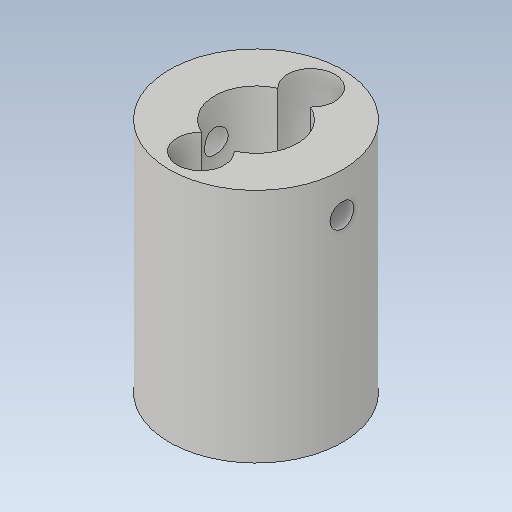
# Autodesk Inventor part: end_effector_connector_arm2_grande
Saved by Autodesk Inventor 2020.1 (Build 241239000, 239)
## iProperties
Created: 2018-02-20
Part Number: end_effector_connector_arm2_grande
Material: Generic
Document SubType Name: Modeling
Designer: Bardo91
Density: 1 g/cm^3
Appearance: Default
Author: Bardo91
Autodesk Inventor part; units mm, degrees
ref_plane "YZ Plane" through (0, 0, 0) normal (1, 0, 0) x (0, 1, 0)
ref_plane "XZ Plane" through (0, 0, 0) normal (0, 1, 0) x (-1, 0, 0)
ref_plane "XY Plane" through (0, 0, 0) normal (0, 0, 1) x (1, 0, 0)
sketch "Boceto5" plane through (0, 0, 0) normal (0, 1, 0) x (-1, 0, 0)
  circle A0 centre (0, 0) radius 11
  line L0 (0, 0) -> (0, -7)
  line L1 (0, 0) -> (0, 7)
  circle A1 centre (0, 7) radius 1.5
  circle A2 centre (0, -7) radius 1.5
  dimension "d25" = 22
  dimension "d26" = 7
  dimension "d27" = 7
  dimension "d28" = 3
  dimension "d29" = 3
  constraints: 4 end point, 3 centre point, 3 coincident, 2 vertical
  measures "d25" diameter of A0
  measures "d26" distance of L0.start L0.end
  measures "d27" distance of L0.start L1.end
  measures "d28" diameter of A1
  measures "d29" diameter of A2
extrude "Extrusión6" add sketch "Boceto5" along normal blind 4
sketch "Boceto6" plane through (0, 4, 0) normal (0, 1, 0) x (1, 0, 0)
  circle A0 centre (0, 0) radius 11
  circle A1 centre (0, -7) radius 1.5 projected
  circle A2 centre (0, -7) radius 3
  circle A3 centre (0, 7) radius 1.5 projected
  circle A4 centre (0, 7) radius 3
  dimension "d32" = 6
  dimension "d33" = 6
  constraints: 3 centre point, 3 coincident
  measures "d32" diameter of A2
  measures "d33" diameter of A4
extrude "Extrusión7" add sketch "Boceto6" along normal blind 8 contours A0
sketch "Boceto7" plane through (0, 12, 0) normal (0, 1, 0) x (1, 0, 0)
  circle A0 centre (0, 0) radius 5.25
  circle A1 centre (0, -7) radius 3 projected
  circle A2 centre (0, -7) radius 3
  circle A3 centre (0, 7) radius 1.5 projected
  circle A4 centre (0, 7) radius 3
  circle A5 centre (0, 0) radius 11
  dimension "d36" = 10.5
  constraints: 4 centre point, 4 coincident
  measures "d36" diameter of A0
extrude "Extrusión8" add sketch "Boceto7" along normal blind 20 contours A5
sketch "Boceto8" plane through (0, 0, 0) normal (1, 0, 0) x (0, 1, 0)
  line L0 (0, 0) -> (23, 0)
  line L1 (23, 0) -> (25, 0)
  circle A0 centre (25, 0) radius 1.5
  dimension "d39" = 23
  dimension "d43" = 2
  dimension "d44" = 3
  constraints: 4 end point, 2 horizontal, 1 centre point, 1 coincident
  measures "d39" distance of L0.start L0.end
  measures "d43" distance of L0.end L1.end
  measures "d44" diameter of A0
extrude "Extrusión10" cut sketch "Boceto8" along normal mid plane 22
move faces "Desplazar2" translate (0, -2, 0) faces at (5.0629, 32, -5.6904)
sketch "Boceto9" plane through (0, 0, 0) normal (0, -1, 0) x (1, 0, 0)
  circle A0 centre (0, 0) radius 3
  dimension "d52" = 6
  constraints: 1 centre point
  measures "d52" diameter of A0
extrude "Extrusión11" cut sketch "Boceto9" against normal blind 12
